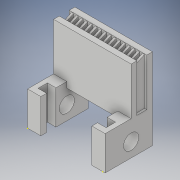
# Autodesk Inventor part: Y Belt Holder
Saved by Autodesk Inventor 2018 (Build 220112000, 112)
## iProperties
Created: 2018-03-14
Part Number: Y Belt Holder
Material: Generic
Document SubType Name: Modeling
Designer: junai
Density: 1 g/cm^3
Appearance: Default
Author: junai
Autodesk Inventor part; units mm, degrees
ref_plane "YZ Plane" through (0, 0, 0) normal (1, 0, 0) x (0, 1, 0)
ref_plane "XZ Plane" through (0, 0, 0) normal (0, 1, 0) x (-1, 0, 0)
ref_plane "XY Plane" through (0, 0, 0) normal (0, 0, 1) x (1, 0, 0)
sketch "Sketch1" plane through (0, 0, 0) normal (0, 1, 0) x (-1, 0, 0)
  point P0 (0, 0)
sketch "Sketch2" plane through (0, 0, 0) normal (0, 1, 0) x (-1, 0, 0)
  line L0 (0, 0) -> (-7, 0)
  line L1 (-7, 0) -> (-7, -25)
  line L2 (-7, -25) -> (0, -25)
  line L3 (0, -25) -> (0, 0)
  line L4 (-7, 0) -> (-34, 0) construction
  line L5 (-34, 0) -> (-41, 0)
  line L6 (-41, 0) -> (-41, -25)
  line L7 (-41, -25) -> (-34, -25)
  line L8 (-34, -25) -> (-34, 0)
  dimension "d0" = 7
  dimension "d1" = 25
  dimension "d2" = 27
  dimension "d3" = 7
  constraints: 18 end point, 4 parallel, 3 horizontal, 2 perpendicular, 1 collinear
  measures "d0" distance of L2.end L1.end
  measures "d1" distance of L0.end L1.end
  measures "d2" distance of L0.end L4.end
  measures "d3" distance of L7.end L6.end
extrude "Extrusion1" add sketch "Sketch2" along normal blind 18
sketch "Sketch3" plane through (0, 18, 0) normal (0, 1, 0) x (1, 0, 0)
  line L0 (7, 0) -> (7, 3) construction
  line L1 (7, 3) -> (2.5, 3)
  line L2 (2.5, 3) -> (2.5, 8)
  line L3 (2.5, 8) -> (7, 8)
  line L4 (7, 8) -> (7, 3)
  line L5 (34, 25) -> (34, 0) projected
  line L6 (34, 3) -> (38.5, 3)
  line L7 (38.5, 3) -> (38.5, 8)
  line L8 (38.5, 8) -> (34, 8)
  line L9 (34, 8) -> (34, 3)
  line L10 (7, 0) -> (7, 25) projected
  point P0 (0, 0)
  dimension "d6" = 3
  dimension "d7" = 4.5
  dimension "d8" = 4.5
  dimension "d9" = 5
  dimension "d10" = 5
  constraints: 18 end point, 4 parallel, 2 collinear, 2 horizontal, 2 perpendicular, 1 point on line
  measures "d6" distance of L0.start L0.end
  measures "d7" distance of L2.end L3.end
  measures "d8" distance of L8.end L7.end
  measures "d9" distance of L3.end L0.end
  measures "d10" distance between parallel lines of L8 L6
sketch "Sketch4" plane through (0, 18, 0) normal (0, 1, 0) x (1, 0, 0)
  line L0 (7, 25) -> (0, 25) projected
  line L1 (41, 0) -> (41, 25) projected
  line L2 (0, 25) -> (41, 25)
  line L3 (41, 25) -> (41, 22)
  line L4 (41, 22) -> (0, 22)
  line L5 (0, 22) -> (0, 25)
  line L6 (34, 25) -> (34, 0) construction
  line L7 (34, 22) -> (34, 16.75) construction
  line L8 (41, 16.75) -> (0, 16.75)
  line L9 (0, 16.75) -> (0, 13.75)
  line L10 (0, 13.75) -> (41, 13.75)
  line L11 (41, 13.75) -> (41, 16.75)
  point P0 (0, 0)
  dimension "d11" = 3
  dimension "d12" = 5.25
  dimension "d13" = 3
  constraints: 18 end point, 6 point on line, 4 parallel, 2 horizontal, 2 perpendicular
  measures "d11" distance between parallel lines of L2 L4
  measures "d12" distance of L7.start L7.end
  measures "d13" distance of L8.end L9.end
extrude "Extrusion2" cut sketch "Sketch3" against normal blind 18
extrude "Extrusion3" add sketch "Sketch4" along normal blind 25
sketch "Sketch5" plane through (41, 0, 0) normal (1, 0, 0) x (0, 0, -1)
  line L0 (0, 18) -> (13.75, 18) projected
  line L1 (25, 0) -> (25, 18) projected
  line L2 (13.75, 18) -> (25, 18)
  line L3 (25, 18) -> (25, 14.9913)
  line L4 (25, 14.9913) -> (13.75, 14.9913)
  line L5 (13.75, 14.9913) -> (13.75, 18)
  point P0 (0, 0)
  constraints: 8 end point, 2 parallel, 1 horizontal, 1 perpendicular, 1 point on line
extrude "Extrusion4" add sketch "Sketch5" against normal up to next
sketch "Sketch6" plane through (41, 0, 0) normal (1, 0, 0) x (0, 0, -1)
  circle A0 centre (13.75, 7.4957) radius 4
  line L0 (25, 0) -> (25, 14.9913) construction
  line L1 (25, 7.4957) -> (13.75, 7.4957) construction
  line L2 (13.75, 18) -> (8, 18) construction
  line L3 (13.75, 18) -> (13.75, 7.4957) construction
  line L4 (13.75, 7.4957) -> (11.75, 7.4957) construction
  point P0 (0, 0)
  dimension "d20" = 8
  dimension "d21" = 2
  constraints: 7 end point, 2 horizontal, 1 centre point, 1 coincident, 1 midpoint, 1 vertical
  measures "d20" diameter of A0
  measures "d21" distance of L1.end L4.end
sketch "Sketch7" plane through (0, 43, 0) normal (0, 1, 0) x (1, 0, 0)
  line L0 (39.8292, 22) -> (38.7292, 22)
  line L1 (38.7292, 22) -> (38.7292, 17.6)
  line L2 (38.7292, 17.6) -> (39.8292, 17.6)
  line L3 (39.8292, 17.6) -> (39.8292, 22)
  line L4 (0, 22) -> (41, 22) projected
  point P0 (0, 0)
  dimension "d22" = 1.1
  dimension "d23" = 4.4
  constraints: 8 end point, 2 parallel, 1 collinear, 1 horizontal, 1 perpendicular
  measures "d22" distance of L2.end L1.end
  measures "d23" distance of L0.end L1.end
extrude "Extrusion5" add sketch "Sketch7" against normal blind 25
sketch "Sketch8" plane through (39.8292, 43, -17.6) normal (1, 0, 0) x (0, 0, -1)
  line L0 (4.4, -25) -> (4.4, 0) projected
  line L1 (0, 0) -> (4.4, 0)
  line L2 (4.4, 0) -> (4.4, -2.3833)
  line L3 (4.4, -2.3833) -> (0, -2.3833)
  line L4 (0, -2.3833) -> (0, 0)
  point P0 (-17.6, -43)
  constraints: 8 end point, 2 parallel, 1 horizontal, 1 perpendicular, 1 point on line
extrude "Extrusion6" cut sketch "Sketch8" against normal blind 25
pattern_linear "Rectangular Pattern1" count 16 spacing 2.5 along (-1, 0, 0) of "Extrusion5"
sketch "Sketch9" plane through (39.8292, 18, -17.6) normal (1, 0, 0) x (0, 0, -1)
  point P0 (-17.6, -18)
sketch "Sketch10" plane through (39.8292, 18, -17.6) normal (1, 0, 0) x (0, 0, -1)
  line L0 (0, 25) -> (0, 0) projected
  line L1 (4.4, 25) -> (4.4, 0) projected
  line L2 (0, 25) -> (4.4, 25)
  line L3 (4.4, 25) -> (4.4, 22.6142)
  line L4 (4.4, 22.6142) -> (0, 22.6142)
  line L5 (0, 22.6142) -> (0, 25)
  point P0 (-17.6, -18)
  constraints: 8 end point, 2 parallel, 1 horizontal, 1 perpendicular, 1 point on line
extrude "Extrusion7" cut sketch "Sketch10" against normal blind 255
draft "FaceDraft1" angle 25 pull direction (0, 0, 1) faces at (39.4626, 40.6142, -20.5333) (36.9626, 40.6142, -20.5333) (34.4626, 40.6142, -20.5333) (31.9626, 40.6142, -20.5333) (29.4626, 40.6142, -20.5333) (26.9626, 40.6142, -20.5333) (24.4626, 40.6142, -20.5333) (21.9626, 40.6142, -20.5333) (19.4626, 40.6142, -20.5333) (16.9626, 40.6142, -20.5333) (14.4626, 40.6142, -20.5333) (11.9626, 40.6142, -20.5333) (9.4626, 40.6142, -20.5333) (6.9626, 40.6142, -20.5333) (4.4626, 40.6142, -20.5333) (1.9626, 40.6142, -20.5333) fixed edges at (39.2792, 40.6142, -17.6) (36.7792, 40.6142, -17.6) (34.2792, 40.6142, -17.6) (31.7792, 40.6142, -17.6) (29.2792, 40.6142, -17.6) (26.7792, 40.6142, -17.6) (24.2792, 40.6142, -17.6) (21.7792, 40.6142, -17.6) (19.2792, 40.6142, -17.6) (16.7792, 40.6142, -17.6) (14.2792, 40.6142, -17.6) (11.7792, 40.6142, -17.6) (9.2792, 40.6142, -17.6) (6.7792, 40.6142, -17.6) (4.2792, 40.6142, -17.6) (1.7792, 40.6142, -17.6)
extrude "Extrusion8" cut sketch "Sketch6" against normal through all
body "Solid1"
